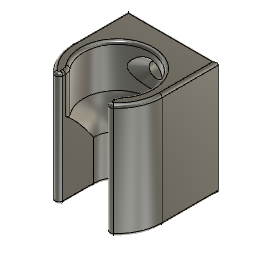
Extension_Bar_Holder (Autodesk Fusion 360 design; units mm, degrees)
Autodesk Fusion 360 part; units mm, degrees
sketch "vertical_profile" plane through (0, 0, 0) normal (0, 0, 1) x (1, 0, 0) in component "Holder"
  line L0 (15.75, 17.75) -> (-15.75, 17.75)
  line L1 (-15.75, 17.75) -> (-15.75, -17.75)
  line L2 (-15.75, -17.75) -> (15.75, -17.75)
  line L3 (15.75, -17.75) -> (15.75, 17.75)
  line L4 (15.75, 17.75) -> (-15.75, -17.75) construction
  line L5 (-15.75, 17.75) -> (15.75, -17.75) construction
  line L6 (0, -17.75) -> (0, -2)
  circle A0 centre (0, -2) radius 11.75
  circle A1 centre (0, -2) radius 8.25
  arc A2 (-15.75, -2) -> (15.75, -2) centre (0, -2) ccw
  dimension "d4" = 31.5
  dimension "d5" = 35.5
  dimension "d6" = 15.75
  dimension "d7" = 23.5
  dimension "d8" = 16.5
  constraint horizontal L0
  constraint perpendicular L0 L1
  constraint parallel L0 L2
  constraint parallel L1 L3
  constraint coincident L4 origin
  constraint coincident L5 origin
  constraint midpoint L2 L6.start
  constraint perpendicular L2 L6
  constraint coincident L6.end A0.centre
  constraint concentric A0 A1
  constraint coincident L3 A2.end
  measures "d4" distance of L1.end L2.end
  measures "d5" distance of L0.end L1.end
  measures "d6" distance of L6.start L6.end
  measures "d7" diameter of A0
  measures "d8" diameter of A1
extrude "Extrude1" add sketch "vertical_profile" along normal blind 40 contours L0 L1 L3 A2 picked at (-0.192182, 15.078616) makes body 1 in component "Holder"
extrude "Extrude2" add sketch "vertical_profile" along normal blind 15 separate body contours A0 picked at (-6.334074, -10.445189) makes body 2 in component "Holder"
sketch "hole_body" plane through (0, 0, 40) normal (0, 0, 1) x (-1, 0, 0) in component "Holder"
  circle A0 centre (0, 2) radius 11.75
  arc A1 (15.75, 2) -> (-15.75, 2) centre (0, 2) ccw
  line L0 (-15.75, 2) -> (-15.75, -17.75)
  line L1 (-15.75, -17.75) -> (15.75, -17.75)
  line L2 (15.75, -17.75) -> (15.75, 2)
  line L3 (0, -17.75) -> (0, -12)
  line L4 (-15.75, -6.25) -> (15.75, -6.25)
  line L5 (15.75, -6.25) -> (15.75, -17.75)
  line L6 (15.75, -17.75) -> (-15.75, -17.75)
  line L7 (-15.75, -17.75) -> (-15.75, -6.25)
  line L8 (-15.75, -6.25) -> (15.75, -17.75) construction
  line L9 (15.75, -6.25) -> (-15.75, -17.75) construction
  point P0 (0, -12)
  dimension "d51" = 5.75
  dimension "d52" = 31.5
  dimension "d53" = 11.5
  constraint midpoint L1 L3.start
  constraint perpendicular L1 L3
  constraint horizontal L4
  constraint perpendicular L4 L5
  constraint parallel L4 L6
  constraint parallel L5 L7
  constraint coincident L8 P0
  constraint coincident L9 P0
  constraint coincident P0 L3.end
  measures "d51" distance of L3.start P0
  measures "d52" distance of L1.end L0.end
  measures "d53" distance of L4.end L1.end
extrude "Extrude6" add sketch "hole_body" against normal blind 15 contours A0 L4 picked at (2.365133, -6.621926) bodies 1 in component "Holder"
sketch "hole_face" plane through (0, 6.25, 0) normal (0, -1, 0) x (1, 0, 0) in component "Holder"
  line L0 (8.3666, 40) -> (-8.3666, 40)
  line L1 (-8.3666, 40) -> (-8.3666, 25)
  line L2 (-8.3666, 25) -> (8.3666, 25)
  line L3 (8.3666, 25) -> (8.3666, 40)
  line L4 (0, 40) -> (0, 32.5)
  dimension "d56" = 7.5
  constraint midpoint L0 L4.start
  constraint perpendicular L0 L4
  measures "d56" distance of L4.start L4.end
hole "Hole2" at (0, 6.25, 32.5) direction (0, 1, 0) diameter 5 depth 11 tip angle 118 countersink diameter 16 countersink angle 90 bodies 1 in component "Holder"
sketch "hole_face_cutout" plane through (0, 0, 40) normal (0, 0, 1) x (-1, 0, 0) in component "Holder"
  arc A0 (8.3666, -6.25) -> (-8.3666, -6.25) centre (0, 2) ccw
  line L0 (-2.783882, -6.25) -> (-8.3666, -6.25)
  arc A1 (15.75, 2) -> (-15.75, 2) centre (0, 2) ccw
  line L1 (-15.75, 2) -> (-15.75, -17.75)
  line L2 (-15.75, -17.75) -> (15.75, -17.75)
  line L3 (15.75, -17.75) -> (15.75, 2)
  line L4 (0, -17.75) -> (0, 2)
  circle A2 centre (0, 2) radius 11.75
  spline S0 degree 2 poles (2.783882, -6.25) (0, -7.21875) (-2.783882, -6.25) knots 0 0 0 0.56568542 0.56568542 0.56568542 weights 1 1.06666667 1
  line L5 (8.3666, -6.25) -> (2.783882, -6.25)
  point P0 (0, -17.75)
  dimension "d62" = 19.75
  dimension "d63" = 23.5
  constraint coincident P0 L4.start
  constraint perpendicular L2 L4
  constraint coincident A0.centre A1.centre
  measures "d62" distance of P0 A0.centre
  measures "d63" diameter of A2
extrude "Extrude7" cut sketch "hole_face_cutout" against normal blind 15 contours L4 A2 S0 L5 | L0 L4 A2 S0 picked at (3.462045, -8.144075) picked at (-3.462045, -8.144075) bodies 1 in component "Holder"
ref_plane "WorkPlane1" through (0, -17.75, 20) normal (0, 1, 0) x (-1, 0, 0) in component "Holder"
ref_plane "WorkPlane2" through (0, -2, 20) normal (0, 1, 0) x (-1, 0, 0) in component "Holder"
sketch "front_cut_out" plane through (0, -17.75, 0) normal (0, 1, 0) x (1, 0, 0) in component "Holder"
  line L0 (-15.25, 0) -> (15.25, 0)
  line L1 (0, 0) -> (0, -20)
  line L2 (8.25, -40) -> (-8.25, -40)
  line L3 (-8.25, -40) -> (-8.25, 0)
  line L4 (-8.25, 0) -> (8.25, 0)
  line L5 (8.25, 0) -> (8.25, -40)
  line L6 (8.25, -40) -> (-8.25, 0) construction
  line L7 (-8.25, -40) -> (8.25, 0) construction
  point P0 (0, -20)
  dimension "d14" = 20
  dimension "d15" = 16.5
  dimension "d16" = 40
  constraint coincident L1.start origin
  constraint perpendicular L0 L1
  constraint horizontal L2
  constraint perpendicular L2 L3
  constraint parallel L2 L4
  constraint parallel L3 L5
  constraint coincident L6 P0
  constraint coincident L7 P0
  constraint coincident P0 L1.end
  measures "d14" distance of L1.start P0
  measures "d15" distance of L3.end L4.end
  measures "d16" distance of L2.end L3.end
sketch "inner_fillet" plane through (0, -2, 20) normal (0, 1, 0) x (1, 0, 0) in component "Holder"
  line L0 (0, 20) -> (-11.75, 20)
  line L1 (-11.75, 20) -> (-11.75, -5)
  line L2 (-11.75, -5) -> (0, -5)
  line L3 (0, -5) -> (0, 20)
  line L4 (-11.75, 20) -> (11.75, 20)
  line L5 (-11.75, -5) -> (-11.75, 5)
  line L6 (-11.75, 5) -> (-8.25, 5)
  arc A0 (-11.75, -5) -> (-8.25, 5) centre (-24.285713, 5) ccw
  line L7 (-8.25, -20) -> (-8.25, 20)
  dimension "d23" = 11.75
  dimension "d24" = 25
  dimension "d26" = 10
  dimension "d27" = 3.5
  constraint horizontal L0
  constraint vertical L1
  constraint horizontal L2
  constraint vertical L3
  constraint perpendicular L2 L5
  constraint perpendicular L5 L6
  constraint tangent A0 L7
  measures "d23" distance of L0.start L0.end
  measures "d24" distance of L0.start L2.end
  measures "d26" distance of L1.end L5.end
  measures "d27" distance of L5.end L6.end
revolve "Revolve2" add sketch "inner_fillet" angle 360 about axis through (0, -2, 0) along (0, 0, -1) contours L1 L5 L6 A0 picked at (-9.465064, 4.282331) bodies 1 2 in component "Holder"
extrude "Extrude5" cut sketch "front_cut_out" along normal blind 15.75 contours L0 L2 L3 L4 L5 picked at (0, -26.666667) bodies 1 in component "Holder"
fillet "Fillet1" radius 1.333333 2 edges at (-8.25, -15.416408, 20) (8.25, -15.416408, 20) on bodies 1 in component "Holder"
fillet "Fillet2" radius 4 2 edges at (-8.25, -10.3666, 32.5) (8.25, -10.3666, 32.5) on bodies 1 in component "Holder"
fillet "Fillet3" radius 1 22 edges at (-15.75, 7.875, 0) (-14.369404, -8.448467, 0) (-9.037431, -13.986787, 0) (-8.25, -7.385165, 0) (0, 6.25, 0) (8.25, -7.385165, 0) (9.037431, -13.986787, 0) (14.369404, -8.448467, 0) (15.75, 7.875, 0) (0, 17.75, 0) (-15.75, 7.875, 40) (-14.369404, -8.448467, 40) (-9.037431, -13.986787, 40) (-8.25, -12.334912, 40) (-8.478764, -10.566162, 40) (0, 9.75, 40) (8.478764, -10.566162, 40) (8.25, -12.334912, 40) (9.037431, -13.986787, 40) (14.369404, -8.448467, 40) (15.75, 7.875, 40) (0, 17.75, 40) on bodies 1 in component "Holder"
component "Holder" placed x (1, 0, 0) y (0, 1, 0) z (0, 0, 1) at (0, 0, 0)
equation "main_shaft_diamater = 16.5 mm"
equation "large_shaft_diameter = 23.5 mm"
equation "wall_thickness = 4 mm"
equation "d4 = large_shaft_diameter + ( 2 * wall_thickness )"
equation "d5 = large_shaft_diameter + ( 3 * wall_thickness )"
equation "d6 = wall_thickness + ( large_shaft_diameter / 2 )"
equation "d7 = large_shaft_diameter"
equation "d8 = main_shaft_diamater"
equation "d9 = height"
equation "height = main_shaft_height + transition_height + large_shaft_height"
equation "d12 = main_shaft_height"
equation "d14 = height / 2"
equation "d15 = main_shaft_diamater"
equation "d16 = height"
equation "d19 = -( large_shaft_diameter + ( 3 * wall_thickness ) )"
equation "d22 = wall_thickness + ( large_shaft_diameter / 2 )"
equation "d23 = large_shaft_diameter / 2"
equation "d24 = main_shaft_height + transition_height"
equation "d26 = transition_height"
equation "d27 = ( large_shaft_diameter - main_shaft_diamater ) / 2"
equation "d30 = wall_thickness + ( large_shaft_diameter / 2 )"
equation "d33 = wall_thickness / 3"
equation "d35 = wall_thickness"
equation "screw_hole_offset = large_shaft_height / 2"
equation "main_shaft_height = 15 mm"
equation "transition_height = 10 mm"
equation "large_shaft_height = 15 mm"
equation "shaft_diameter_differentce = ( large_shaft_diameter - main_shaft_diamater ) / 2"
equation "d51 = ( ( 2 * wall_thickness ) + shaft_diameter_differentce ) / 2"
equation "d52 = ( 2 * wall_thickness ) + large_shaft_diameter"
equation "d53 = ( 2 * wall_thickness ) + shaft_diameter_differentce"
equation "d54 = -large_shaft_height"
equation "d56 = screw_hole_offset"
equation "d62 = ( 2 * wall_thickness ) + ( large_shaft_diameter / 2 )"
equation "d63 = large_shaft_diameter"
equation "d64 = -main_shaft_height"
